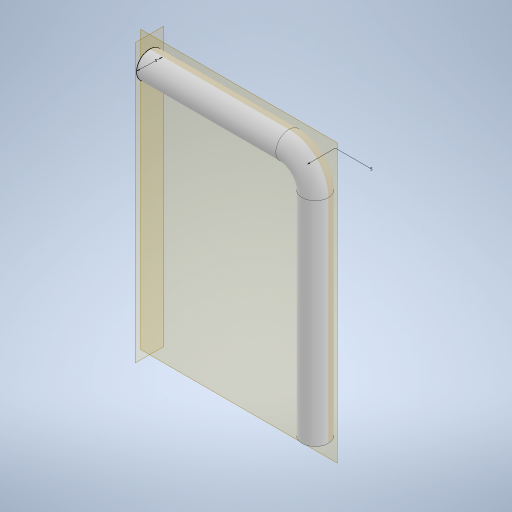
# Autodesk Inventor part: трубка ветка
Saved by Autodesk Inventor 2023 (Build 270158000, 158)
## iProperties
Created: 2024-01-16
Part Number: трубка ветка
Material: Типовые
Document SubType Name: Modeling
Designer: liza
Density: 1 g/cm^3
Appearance: По умолчанию
Author: liza
Autodesk Inventor part; units mm, degrees
ref_plane "XZ Plane" through (0, 0, 0) normal (0, 1, 0) x (-1, 0, 0)
sketch "Эскиз1" plane through (0, 0, 0) normal (1, 0, 0) x (0, 1, 0)
  circle A0 centre (0, 0) radius 2.5
  dimension "d0" = 5
  constraints: 1 centre point, 1 coincident
  measures "d0" diameter of A0
sketch3d "3D эскиз2"
  line L0 (0, 0, 0) -> (26.574, 0, 0)
  arc A0 (26.574, 0, 0) -> (31.574, -5, 0) centre (26.574, -5, 0) ccw
  line L1 (31.574, -5, 0) -> (31.574, -45.5693, 0)
  dimension "d13" = 5
sweep "Сдвиг2" add profiles "Эскиз1" path "3D эскиз2"
sketch3d "3D эскиз1"
